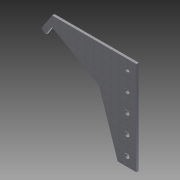
# Autodesk Inventor part: grabber_plate_metal_hook_long
Saved by Autodesk Inventor 2011 (Build 150239000, 239)
## iProperties
Created: 2013-01-17
Part Number: grabber_plate_metal_hook_long
Document SubType Name: Modeling
Designer: Christopher
Density: 1 g/cm^3
Author: Christopher
Autodesk Inventor part; units mm, degrees
ref_plane "YZ Plane" through (0, 0, 0) normal (1, 0, 0) x (0, 1, 0)
ref_plane "XZ Plane" through (0, 0, 0) normal (0, 1, 0) x (-1, 0, 0)
ref_plane "XY Plane" through (0, 0, 0) normal (0, 0, 1) x (1, 0, 0)
sketch "Sketch1" plane through (0, 0, 0) normal (0, 0, 1) x (1, 0, 0)
  line L0 (128.0664, -77.27) -> (153.4664, -77.27)
  line L1 (153.4664, 49.73) -> (153.4664, -77.27)
  line L2 (102.6664, -0.6801) -> (39.1664, 35.7867)
  line L3 (39.1664, 35.7867) -> (30.7882, 23.0867)
  line L4 (30.7882, 23.0867) -> (24.3791, 27.3148)
  line L5 (24.3791, 27.3148) -> (39.1664, 49.73)
  line L6 (153.4664, 49.73) -> (39.1664, 49.73)
  line L7 (128.0664, -77.27) -> (102.6664, -0.6801)
  point P0 (0, 0)
  point P1 (140.7664, -39.17)
  point P2 (140.7664, -64.57)
  point P3 (140.7664, -13.77)
  point P4 (140.7664, 11.63)
  point P5 (140.7664, 37.03)
  dimension "d10" = 25.4
  dimension "d11" = 12.7
  dimension "d29" = 127
  dimension "d34" = 12.7
  dimension "d35" = 63.5
  dimension "d36" = 12.7
  dimension "d37" = 25.4
  dimension "d38" = 25.4
  dimension "d39" = 25.4
  dimension "d40" = 25.4
  dimension "d41" = 114.3
  constraints: 16 end point, 4 perpendicular, 4 vertical alignment, 1 horizontal
  measures "d10" distance of point (140.766, -64.57) point (140.766, -39.17)
  measures "d11" distance from line of L0 point (140.766, -64.57)
  measures "d29" distance of L1.start L0.end
  measures "d34" vertical distance of L2.end L3.end
  measures "d35" horizontal distance of L2.start L2.end
  measures "d36" distance from line of L1 point (140.766, -64.57)
  measures "d37" distance of L0.start L0.end
  measures "d38" distance of point (140.766, -39.17) point (140.766, -13.77)
  measures "d39" distance of point (140.766, 11.63) point (140.766, -13.77)
  measures "d40" distance of point (140.766, 37.03) point (140.766, 11.63)
  measures "d41" distance of L1.start L5.end
extrude "Extrusion1" add sketch "Sketch1" against normal blind 3.175
hole "Hole1" at (140.7664, -39.17, 0) at (140.7664, -64.57, 0) at (140.7664, -13.77, 0) at (140.7664, 11.63, 0) at (140.7664, 37.03, 0) direction (0, 0, -1) diameter 6.35 depth 25.4 tip angle 118
fillet "Fillet1" radius 12.7 1 edges at (102.6664, -0.6801, -1.5875)
body "Solid1"
